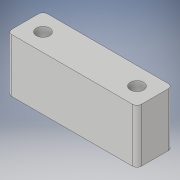
# Autodesk Inventor part: Bearing Seat 8mm
Saved by Autodesk Inventor 2019 (Build 230136000, 136)
## iProperties
Created: 2019-11-28
Part Number: Bearing Seat 8mm
Material: Generic
Document SubType Name: Modeling
Designer: micha
Density: 1 g/cm^3
Appearance: Default
Author: micha
Autodesk Inventor part; units mm, degrees
ref_plane "YZ Plane" through (0, 0, 0) normal (1, 0, 0) x (0, 1, 0)
ref_plane "XZ Plane" through (0, 0, 0) normal (0, 1, 0) x (-1, 0, 0)
ref_plane "XY Plane" through (0, 0, 0) normal (0, 0, 1) x (1, 0, 0)
sketch "Sketch1" plane through (0, 0, 0) normal (0, 1, 0) x (-1, 0, 0)
  line L0 (0, 0) -> (42, 0)
  circle A0 centre (42, 0) radius 3
  circle A1 centre (0, 0) radius 3
  line L1 (0, 0) -> (-8, 0)
  line L2 (-8, 0) -> (-8, -8)
  line L3 (42, 0) -> (42, 8)
  line L4 (42, 8) -> (50, 8)
  line L5 (50, 8) -> (-8, 8)
  line L6 (-8, 8) -> (-8, -8)
  line L7 (-8, -8) -> (50, -8)
  line L8 (50, -8) -> (50, 8)
  dimension "d0" = 42
  dimension "d1" = 6
  dimension "d2" = 6
  dimension "d3" = 8
  dimension "d4" = 8
  dimension "d5" = 8
  dimension "d6" = 8
  constraints: 18 end point, 4 perpendicular, 3 horizontal, 2 centre point, 2 coincident, 2 parallel
  measures "d0" distance of L0.start L0.end
  measures "d1" diameter of A0
  measures "d2" diameter of A1
  measures "d3" distance of L1.start L1.end
  measures "d4" distance of L1.end L2.end
  measures "d5" distance of L3.start L3.end
  measures "d6" distance of L3.end L4.end
extrude "Extrusion1" add sketch "Sketch1" along normal blind 24 contours A1 L1 L6 L5 L3 A0 L0 | L0 A0 L3 L4 L8 L7 L2 L1 A1
fillet "Fillet1" radius 2 4 edges at (8, 12, 8) (8, 12, -8) (-50, 12, 8) (-50, 12, -8)
body "Solid1"
